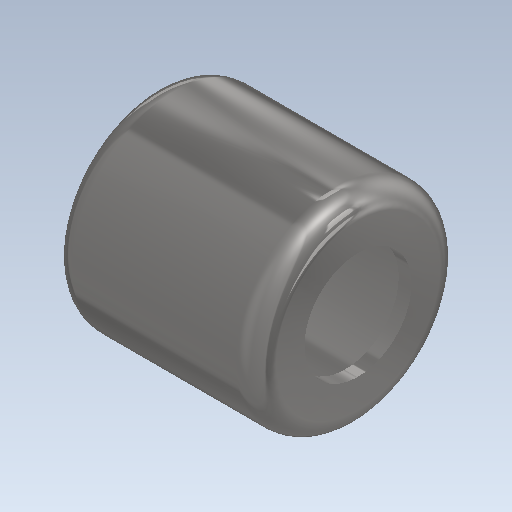
# Autodesk Inventor part: HK0408FT2SH
Saved by Autodesk Inventor 2021.3 (Build 253353010, 353A)
## iProperties
Category: PARTsolutions
Company: NTN
Part Number: HK0408FT2SH
Material: 一般
Catalog Web Link: www.cadenas.de
Description: Needle Roller Shell Bearings open-ended SH-
Vendor: NTN
Document SubType Name: Modeling
Designer: partserver
Manufacturer: NTN
Mass: 0.113116 g
Surface Area: 4.66705 cm^2
Volume: 0.113116 cm^3
Density: 1 g/cm^3
Appearance: ステンレス - ブラシ仕上げ
PSOL_IDENT_0: {$CADENAS_DATA\23d-libs\ntn\needle_roler_bearings\needle_roller_shell_bearings_open_ended.prj},198 {
PSOL_IDENT_1: VTYP=3D},{NB=HK0408FT2SH},{LINA=HK0408FT2SH},{NN=Needle Roller Shell Bearings open-ended SH},{DATE=2
PSOL_IDENT_2: 3.10.2020 01:12:36},{GEOMDATE=20.04.2020 08:31:59},{VERSION=},{LINEID=20},{WBVAR=},{WBNUMERIC=}  {NB=
PSOL_IDENT_3: HK0408FT2SH},{LINA=HK0408FT2SH},{KT=DUMMY},{FW=4},{D=8.0},{C=8},{ORDER=HK0408FT2},{CR=1770},{COR=127
PSOL_IDENT_4: 0},{CRF=180},{CORF=129},{LSG=30000},{LSO=45000},{MASS=0.0016},{IT=-},{RT=1.6},{VER=1},{T=0.500},{DW=
PSOL_IDENT_5: 1.500},{LW=4.000},{NR=6.000},{CID=4.750},{CD=6.250},{CW=6.600},{SD=4.200}
NB: HK0408FT2SH
NN: Needle Roller Shell Bearings open-ended SH
NBSYN: $ORDER.SH
LINA: HK0408FT2SH
CATALOG: NTN Corporation
FW: 4
D: 8
C: 8
ORDER: HK0408FT2
CR: 1770
COR: 1270
CRF: 180
CORF: 129
LSG: 30000
LSO: 45000
MASS: 0.0016
IT: -
SUPPLIER: NTN
ARTICLENO: HK0408FT2SH
BOMINFO: HK0408FT2SH
CREATOR: CADENAS GmbH
d1: 0.000 mm
Title: HK0408FT2SH
Author: Cadenas PARTsolutions
Autodesk Inventor part; units mm, degrees
sketch "Sketch_1" plane through (0, 0, 0) normal (0, 0, 1) x (1, 0, 0)
  line L0 (8, 0) -> (0, 0)
  line L1 (0, 2.1) -> (0.5, 2.1)
  line L2 (0.5, 2.1) -> (0.5, 3.2)
  arc A0 (0.8, 3.5) -> (0.5, 3.2) centre (0.8, 3.2) ccw
  line L3 (0.8, 3.5) -> (7.2, 3.5)
  arc A1 (7.5, 3.2) -> (7.2, 3.5) centre (7.2, 3.2) ccw
  line L4 (7.5, 3.2) -> (7.5, 2.1)
  line L5 (7.5, 2.1) -> (8, 2.1)
  line L6 (8, 2.1) -> (8, 3.2)
  arc A2 (8, 3.2) -> (7.2, 4) centre (7.2, 3.2) ccw
  line L7 (7.2, 4) -> (0.8, 4)
  arc A3 (0.8, 4) -> (0, 3.2) centre (0.8, 3.2) ccw
  line L8 (0, 3.2) -> (0, 2.1)
  constraints: 18 end point, 8 point on circle, 4 centre point
revolve "Revolution1" add sketch "Sketch_1" angle 360 about axis through (8, 0, 0) along (1, 0, 0)
ref_plane "IP_1_XY" through (0, 0, 0) normal (1, 0, 0) x (0, 0, -1)
ref_plane "IP_1_YZ" through (0, 0, 0) normal (0, 0, -1) x (0, 1, 0)
ref_plane "IP_1_ZX" through (0, 0, 0) normal (0, 1, 0) x (1, 0, 0)
ref_plane "IP_5_XY" through (4, 0, 0) normal (1, 0, 0) x (0, 0, -1)
ref_plane "IP_5_YZ" through (4, 0, 0) normal (0, 0, -1) x (0, 1, 0)
ref_plane "IP_5_ZX" through (4, 0, 0) normal (0, 1, 0) x (1, 0, 0)
ref_plane "IP_6_XY" through (5.6, 0, 0) normal (1, 0, 0) x (0, 0, -1)
ref_plane "IP_6_YZ" through (5.6, 0, 0) normal (0, 0, -1) x (0, 1, 0)
ref_plane "IP_6_ZX" through (5.6, 0, 0) normal (0, 1, 0) x (1, 0, 0)
body "Solid1"
